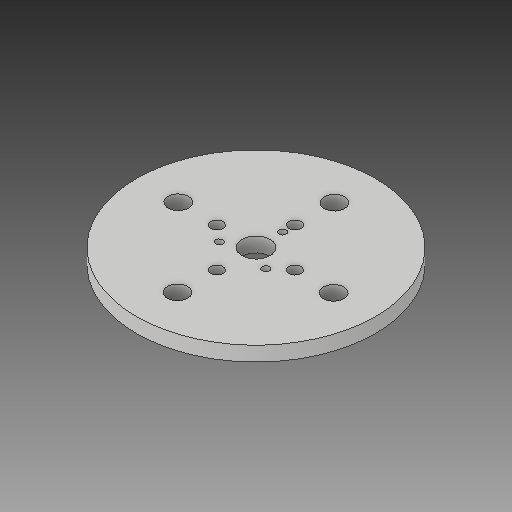
# Autodesk Inventor part: КВ33.044.405 -  Боковина шкива
Saved by Autodesk Inventor 2019 (Build 230136000, 136)
## iProperties
Created: 2019-08-06
Part Number: КВ33.044.405 -  Боковина шкива
Material: Типовые
Document SubType Name: Modeling
Designer: Петров Иван
Density: 1 g/cm^3
Appearance: По умолчанию
Mass: 5.3369 g
Surface Area: 43.6941 cm^2
Volume: 5.3369 cm^3
Author: Петров Иван
Autodesk Inventor part; units mm, degrees
ref_plane "YZ Plane" through (0, 0, 0) normal (1, 0, 0) x (0, 1, 0)
ref_plane "XZ Plane" through (0, 0, 0) normal (0, 1, 0) x (-1, 0, 0)
ref_plane "XY Plane" through (0, 0, 0) normal (0, 0, 1) x (1, 0, 0)
sketch "Эскиз1" plane through (0, 0, 0) normal (0, 1, 0) x (-1, 0, 0)
  arc A0 (-0.25, 9.2247) -> (0.25, 9.2247) centre (0, 8) ccw
  line L0 (-0.25, 10.9972) -> (-0.25, 9.2247)
  arc A1 (-0.25, 10.9972) -> (-1.1469, -10.94) centre (0, 0) ccw
  line L1 (-1.1469, -10.6297) -> (-1.1469, -10.94)
  line L2 (-0.8473, -10.6297) -> (-1.1469, -10.6297)
  line L3 (-0.8473, -10.9673) -> (-0.8473, -10.6297)
  arc A2 (-0.8473, -10.9673) -> (0.8535, -10.9668) centre (0, 0) ccw
  line L4 (0.8535, -10.6297) -> (0.8535, -10.9668)
  line L5 (1.1541, -10.6297) -> (0.8535, -10.6297)
  line L6 (1.1541, -10.9393) -> (1.1541, -10.6297)
  arc A3 (1.1541, -10.9393) -> (0.25, 10.9972) centre (0, 0) ccw
  line L7 (0.25, 9.2247) -> (0.25, 10.9972)
  circle A4 centre (8, 0) radius 1.25
  circle A5 centre (0, -8) radius 1.25
  circle A6 centre (-8, 0) radius 1.25
  circle A7 centre (0, -5.5) radius 0.75
  circle A8 centre (4.7631, 2.75) radius 0.75
  circle A9 centre (-4.7631, 2.75) radius 0.75
  circle A10 centre (0, 0) radius 2.9
  arc A11 (0.25, 9.2247) -> (-0.25, 9.2247) centre (0, 8) ccw
  circle A12 centre (0, 0) radius 22.5
  point P0 (0, 0)
  dimension "d8" = 45
  constraints: 16 end point, 13 centre point, 10 point on circle, 1 coincident
  measures "d8" diameter of A12
extrude "Выдавливание1" add sketch "Эскиз1" along normal blind 3 contours A0 L7 A3 L6 L5 L4 A2 L3 L2 L1 A1 L0 | A12
sketch "Эскиз2" plane through (0, 3, 0) normal (0, 1, 0) x (1, 0, 0)
  arc A0 (-14.8717, -1.6857) -> (-18.0997, 0.0968) centre (-15.9998, 0.0856) ccw
  arc A1 (-6.8718, -1.7285) -> (-9.1468, -1.7163) centre (-7.9999, 0.0428) ccw
  circle A2 centre (0, 0) radius 4
  arc A3 (-1.7285, 6.8718) -> (-1.7163, 9.1468) centre (0.0428, 7.9999) ccw
  arc A4 (-1.6857, 14.8717) -> (0.0968, 18.0997) centre (0.0856, 15.9998) ccw
  arc A5 (6.8718, 1.7285) -> (9.1468, 1.7163) centre (7.9999, -0.0428) ccw
  arc A6 (14.8717, 1.6857) -> (18.0997, -0.0968) centre (15.9998, -0.0856) ccw
  arc A7 (1.7285, -6.8718) -> (1.7163, -9.1468) centre (-0.0428, -7.9999) ccw
  arc A8 (1.6857, -14.8717) -> (-0.0968, -18.0997) centre (-0.0856, -15.9998) ccw
  circle A9 centre (-15.9998, 0.0856) radius 2.1
  circle A10 centre (-7.9999, 0.0428) radius 2.1
  circle A11 centre (0, 0) radius 4
  circle A12 centre (0.0428, 7.9999) radius 2.1
  circle A13 centre (0.0856, 15.9998) radius 2.1
  circle A14 centre (7.9999, -0.0428) radius 2.1
  circle A15 centre (15.9998, -0.0856) radius 2.1
  circle A16 centre (-0.0428, -7.9999) radius 2.1
  circle A17 centre (-0.0856, -15.9998) radius 2.1
  dimension "d4" = 4.2
  constraints: 18 centre point, 16 point on circle, 9 coincident, 4 concentric
  measures "d4" diameter of A14
extrude "Выдавливание2" cut sketch "Эскиз2" against normal blind 10 contours A9 A0 | A13 A4 | A15 A6 | A17 A8
offset faces "Размер1" outward 2 faces at (-22.427, 2, -1.8105)
sketch "Эскиз3" plane through (0, 3, 0) normal (0, 1, 0) x (1, 0, 0)
  circle A0 centre (15.9998, -0.0856) radius 2.1 projected
  circle A1 centre (-15.9998, 0.0856) radius 2.1 projected
  circle A2 centre (0.0856, 15.9998) radius 2.1 projected
  circle A3 centre (-0.0856, -15.9998) radius 2.1 projected
  circle A4 centre (0, 0) radius 2.9 projected
  circle A5 centre (8, 0) radius 1.25 projected
  circle A6 centre (0, 8) radius 1.25 projected
  circle A7 centre (-8, 0) radius 1.25 projected
  circle A8 centre (4.7631, -2.75) radius 0.75 projected
  circle A9 centre (-4.7631, -2.75) radius 0.75 projected
  circle A10 centre (0, 5.5) radius 0.75 projected
  circle A11 centre (0, -8) radius 1.25 projected
  circle A12 centre (0, 0) radius 24.5 projected
